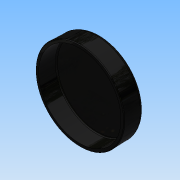
# Autodesk Inventor part: Signal_tower_E
Saved by Autodesk Inventor 2017.3 (Build 213256000, 256)
## iProperties
Created: 2017-03-21
Part Number: Signal_tower_E
Material: PC/ABS plast
Document SubType Name: Modeling
Designer: CAD
Mass: 5.06476 g
Surface Area: 135.125 cm^2
Volume: 14.1762 cm^3
Density: 0.357273 g/cm^3
Appearance: Železo – černá
Stock Number: SIEMENS
Hmotnost: 0
Hotovo: 0
Objem: 0
X: 0
Y: 0
Z: 0
Author: CAD
Autodesk Inventor part; units mm, degrees
ref_plane "YZ Plane" through (0, 0, 0) normal (1, 0, 0) x (0, 1, 0)
ref_plane "XZ Plane" through (0, 0, 0) normal (0, 1, 0) x (-1, 0, 0)
ref_plane "XY Plane" through (0, 0, 0) normal (0, 0, 1) x (1, 0, 0)
sketch "Náčrt2" plane through (0, 0, 0) normal (0, 0, 1) x (1, 0, 0)
  line L0 (-32.5, 0) -> (-35, 0)
  line L1 (0, 0) -> (0, 13.9077) construction
  line L2 (-32.5, 0) -> (0, 0) construction
  line L3 (-35, 0) -> (-34.5908, 13.0937)
  line L4 (-31.5923, 16) -> (0, 16)
  arc A0 (-31.5923, 16) -> (-34.5908, 13.0937) centre (-31.5923, 13) ccw
  line L5 (-32.5, 0) -> (-32.5, 13)
  arc A1 (-31.5923, 13.9077) -> (-32.5, 13) centre (-31.5923, 13) ccw
  line L6 (-31.5923, 13.9077) -> (0, 13.9077)
  line L7 (0, 13.9077) -> (0, 16)
  point P0 (-34.5, 16)
  dimension "d27" = 70
  dimension "d28" = 16
  dimension "d29" = 69
  dimension "d30" = 3
  dimension "d31" = 65
  constraints: 16 end point, 4 point on circle, 4 tangent, 2 centre point, 2 horizontal, 2 point on line, 2 vertical, 1 coincident, 1 parallel, 1 perpendicular
  measures "d27" diameter of L0.end L1
  measures "d28" distance between parallel lines of L0 L4
  measures "d29" diameter of point (-34.5, 16) L1
  measures "d30" radius of A0
  measures "d31" diameter of L5 L1
revolve "Rotace3" add sketch "Náčrt2" angle 360 about axis through (0, 0, 0) along (0, 1, 0)
chamfer "Zkosení1" distance 0.5 angle 45 1 edges at (35, 0, 0)
